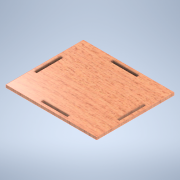
# Autodesk Inventor part: Top_100wx100d
Saved by Autodesk Inventor 2022.2 (Build 262287000, 287)
## iProperties
Created: 2023-04-17
Part Number: Top_100wx100d
Material: Wood (Oak)
Document SubType Name: Modeling
Designer: jaege
Density: 0.76 g/cm^3
Appearance: Red Oak - Natural Low Gloss
Author: jaege
Autodesk Inventor part; units mm, degrees
ref_plane "YZ Plane" through (0, 0, 0) normal (1, 0, 0) x (0, 1, 0)
ref_plane "XZ Plane" through (0, 0, 0) normal (0, 1, 0) x (-1, 0, 0)
ref_plane "XY Plane" through (0, 0, 0) normal (0, 0, 1) x (1, 0, 0)
sketch "Sketch1" plane through (0, 0, 0) normal (0, 1, 0) x (-1, 0, 0)
  line L0 (60, -50) -> (-60, -50) construction
  line L1 (-60, -50) -> (-60, 50) construction
  line L2 (-60, 50) -> (60, 50) construction
  line L3 (60, 50) -> (60, -50) construction
  line L4 (64, -54) -> (-64, -54) construction
  line L5 (-64, -54) -> (-64, 54) construction
  line L6 (-64, 54) -> (64, 54) construction
  line L7 (64, 54) -> (64, -54) construction
  line L8 (68, -58) -> (-68, -58)
  line L9 (-68, -58) -> (-68, 58)
  line L10 (-68, 58) -> (68, 58)
  line L11 (68, 58) -> (68, -58)
  line L12 (64, -20) -> (60, -20)
  line L13 (60, -20) -> (60, 20)
  line L14 (60, 20) -> (64, 20)
  line L15 (64, 20) -> (64, -20)
  line L16 (-60, 20) -> (-64, 20)
  line L17 (-64, 20) -> (-64, -20)
  line L18 (-64, -20) -> (-60, -20)
  line L19 (-60, -20) -> (-60, 20)
  line L20 (-20, -50) -> (20, -50)
  line L21 (20, -50) -> (20, -54)
  line L22 (20, -54) -> (-20, -54)
  line L23 (-20, -54) -> (-20, -50)
  line L24 (20, 50) -> (-20, 50)
  line L25 (-20, 50) -> (-20, 54)
  line L26 (-20, 54) -> (20, 54)
  line L27 (20, 54) -> (20, 50)
  point P0 (0, 0)
  point P1 (0, -50)
  point P2 (60, 0)
  point P3 (60, 0)
  point P4 (0, -50)
  point P5 (62, 20)
  point P6 (62, -20)
  dimension "d0" = 4
  dimension "d1" = 4
  dimension "d2" = 120
  dimension "d3" = 100
  dimension "d4" = 40
  constraints: 56 end point, 14 parallel, 12 point on line, 8 perpendicular, 6 midpoint, 5 horizontal, 2 horizontal alignment, 2 vertical alignment, 6 other
  measures "d0" distance between parallel lines of L3 L7
  measures "d1" distance between parallel lines of L7 L11
  measures "d2" distance between parallel lines of L1 L3
  measures "d3" distance between parallel lines of L2 L0
  measures "d4" distance of point (62, 20) point (62, -20)
extrude "Extrusion1" add sketch "Sketch1" along normal blind 4
body "Solid1"
